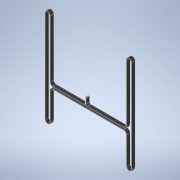
# Autodesk Inventor part: GT2 Belt
Saved by Autodesk Inventor 2022 (Build 260153000, 153)
## iProperties
Created: 2022-06-12
Part Number: GT2 Belt
Material: Generic
Document SubType Name: Modeling
Designer: Nick
Density: 1 g/cm^3
Appearance: Default
Author: Nick
Autodesk Inventor part; units mm, degrees
ref_plane "YZ Plane" through (0, 0, 0) normal (1, 0, 0) x (0, 1, 0)
ref_plane "Work Plane1" through (-134.6469, -237.4299, -822.9431) normal (0, 0, -1) x (0, -1, 0)
ref_plane "Work Plane3" through (-210.2684, -168.4601, -822.9431) normal (0, 1, 0) x (-1, 0, 0)
sketch "Sketch3" plane through (-210.2684, -168.4601, -822.9431) normal (0, 1, 0) x (-1, 0, 0)
  line L0 (0, 0) -> (1, 0)
  line L1 (1, 0) -> (1, -6)
  line L2 (1, -6) -> (0, -6)
  line L3 (0, -6) -> (0, 0)
  point P0 (-210.2684, 822.9431)
  dimension "d10" = 1
  dimension "d11" = 6
  constraints: 8 end point, 2 parallel, 1 horizontal, 1 perpendicular
  measures "d10" distance of L1.end L2.end
  measures "d11" distance of L0.end L1.end
sketch "Sketch1" plane through (-134.6469, -237.4299, -822.9431) normal (0, 0, -1) x (0, -1, 0)
  line L0 (0, 4.84) -> (-47.9698, 4.84)
  line L1 (-52.6298, 9.5) -> (-52.6298, 134.5)
  line L2 (-57.3098, 134.5) -> (-57.3098, 79.9614)
  line L3 (-57.3098, 73.4614) -> (-57.3098, 9.5)
  line L4 (-163, 4.84) -> (-61.9698, 4.84)
  line L5 (-163, -4.84) -> (0, -4.84)
  circle A0 centre (-61.9698, 9.5) radius 4.5 construction
  circle A1 centre (-47.9698, 9.5) radius 4.5 construction
  circle A2 centre (-61.9698, 134.5) radius 4.5
  circle A3 centre (-47.9698, 134.5) radius 4.5
  circle A4 centre (-163, 0) radius 4.5 construction
  circle A5 centre (-163, 144) radius 4.5
  arc A6 (1.9272, 148.2347) -> (2.8669, 147.6644) centre (2.3867, 147.9324) ccw construction
  arc A7 (3.1094, 147.709) -> (2.8669, 147.6644) centre (3.0067, 147.5864) ccw construction
  arc A8 (3.4244, 147.4203) -> (3.1094, 147.709) centre (0, 144) ccw construction
  arc A9 (3.4011, 147.1749) -> (3.4244, 147.4203) centre (3.3112, 147.3073) ccw construction
  arc A10 (3.4011, 147.1749) -> (4.051, 146.2883) centre (3.7099, 146.7197) ccw construction
  arc A11 (4.2921, 146.2368) -> (4.051, 146.2883) centre (4.1503, 146.1628) ccw construction
  arc A12 (4.4727, 145.8495) -> (4.2921, 146.2368) centre (0, 144) ccw construction
  arc A13 (4.3571, 145.6317) -> (4.4727, 145.8495) centre (4.3248, 145.7884) ccw construction
  arc A14 (4.3571, 145.6317) -> (4.6183, 144.5639) centre (4.4683, 145.093) ccw construction
  arc A15 (4.8214, 144.424) -> (4.6183, 144.5639) centre (4.662, 144.41) ccw construction
  arc A16 (4.84, 143.9971) -> (4.8214, 144.424) centre (0, 144) ccw construction
  arc A17 (4.6499, 143.8401) -> (4.84, 143.9971) centre (4.68, 143.9972) ccw construction
  arc A18 (4.6499, 143.8401) -> (4.4826, 142.7536) centre (4.5464, 143.2999) ccw construction
  arc A19 (4.6166, 142.5466) -> (4.4826, 142.7536) centre (4.464, 142.5947) ccw construction
  arc A20 (4.4705, 142.1451) -> (4.6166, 142.5466) centre (0, 144) ccw construction
  arc A21 (4.2347, 142.0728) -> (4.4705, 142.1451) centre (4.3227, 142.2065) ccw construction
  arc A22 (4.2347, 142.0728) -> (3.6644, 141.1331) centre (3.9324, 141.6133) ccw construction
  arc A23 (3.709, 140.8906) -> (3.6644, 141.1331) centre (3.5864, 140.9933) ccw construction
  arc A24 (3.4203, 140.5756) -> (3.709, 140.8906) centre (0, 144) ccw construction
  arc A25 (3.1749, 140.5989) -> (3.4203, 140.5756) centre (3.3073, 140.6888) ccw construction
  arc A26 (3.1749, 140.5989) -> (2.2883, 139.949) centre (2.7197, 140.2901) ccw construction
  arc A27 (2.2368, 139.7079) -> (2.2883, 139.949) centre (2.1628, 139.8497) ccw construction
  arc A28 (1.8495, 139.5273) -> (2.2368, 139.7079) centre (0, 144) ccw construction
  arc A29 (1.6317, 139.6429) -> (1.8495, 139.5273) centre (1.7884, 139.6752) ccw construction
  arc A30 (1.6317, 139.6429) -> (0.5639, 139.3817) centre (1.093, 139.5317) ccw construction
  arc A31 (0.424, 139.1786) -> (0.5639, 139.3817) centre (0.41, 139.338) ccw construction
  arc A32 (-0.0029, 139.16) -> (0.424, 139.1786) centre (0, 144) ccw construction
  arc A33 (-0.1599, 139.3501) -> (-0.0029, 139.16) centre (-0.0028, 139.32) ccw construction
  arc A34 (-0.1599, 139.3501) -> (-1.2464, 139.5174) centre (-0.7001, 139.4536) ccw construction
  arc A35 (-1.4534, 139.3834) -> (-1.2464, 139.5174) centre (-1.4053, 139.536) ccw construction
  arc A36 (-1.8549, 139.5295) -> (-1.4534, 139.3834) centre (0, 144) ccw construction
  arc A37 (-1.9272, 139.7653) -> (-1.8549, 139.5295) centre (-1.7935, 139.6773) ccw construction
  arc A38 (-1.9272, 139.7653) -> (-2.8669, 140.3356) centre (-2.3867, 140.0676) ccw construction
  arc A39 (-3.1094, 140.291) -> (-2.8669, 140.3356) centre (-3.0067, 140.4136) ccw construction
  arc A40 (-3.4244, 140.5797) -> (-3.1094, 140.291) centre (0, 144) ccw construction
  arc A41 (-3.4011, 140.8251) -> (-3.4244, 140.5797) centre (-3.3112, 140.6927) ccw construction
  arc A42 (-3.4011, 140.8251) -> (-4.051, 141.7117) centre (-3.7099, 141.2803) ccw construction
  arc A43 (-4.2921, 141.7632) -> (-4.051, 141.7117) centre (-4.1503, 141.8372) ccw construction
  arc A44 (-4.4727, 142.1505) -> (-4.2921, 141.7632) centre (0, 144) ccw construction
  arc A45 (-4.3571, 142.3683) -> (-4.4727, 142.1505) centre (-4.3248, 142.2116) ccw construction
  arc A46 (-4.3571, 142.3683) -> (-4.6183, 143.4361) centre (-4.4683, 142.907) ccw construction
  arc A47 (-4.8214, 143.576) -> (-4.6183, 143.4361) centre (-4.662, 143.59) ccw construction
  arc A48 (-4.84, 144.0029) -> (-4.8214, 143.576) centre (0, 144) ccw construction
  arc A49 (-4.6499, 144.1599) -> (-4.84, 144.0029) centre (-4.68, 144.0028) ccw construction
  arc A50 (-4.6499, 144.1599) -> (-4.4826, 145.2464) centre (-4.5464, 144.7001) ccw construction
  arc A51 (-4.6166, 145.4534) -> (-4.4826, 145.2464) centre (-4.464, 145.4053) ccw construction
  arc A52 (-4.4705, 145.8549) -> (-4.6166, 145.4534) centre (0, 144) ccw construction
  arc A53 (-4.2347, 145.9272) -> (-4.4705, 145.8549) centre (-4.3227, 145.7935) ccw construction
  arc A54 (-4.2347, 145.9272) -> (-3.6644, 146.8669) centre (-3.9324, 146.3867) ccw construction
  arc A55 (-3.709, 147.1094) -> (-3.6644, 146.8669) centre (-3.5864, 147.0067) ccw construction
  arc A56 (-3.4203, 147.4244) -> (-3.709, 147.1094) centre (0, 144) ccw construction
  arc A57 (-3.1749, 147.4011) -> (-3.4203, 147.4244) centre (-3.3073, 147.3112) ccw construction
  arc A58 (-3.1749, 147.4011) -> (-2.2883, 148.051) centre (-2.7197, 147.7099) ccw construction
  arc A59 (-2.2368, 148.2921) -> (-2.2883, 148.051) centre (-2.1628, 148.1503) ccw construction
  arc A60 (-1.8495, 148.4727) -> (-2.2368, 148.2921) centre (0, 144) ccw construction
  arc A61 (-1.6317, 148.3571) -> (-1.8495, 148.4727) centre (-1.7884, 148.3248) ccw construction
  arc A62 (-1.6317, 148.3571) -> (-0.5639, 148.6183) centre (-1.093, 148.4683) ccw construction
  arc A63 (-0.424, 148.8214) -> (-0.5639, 148.6183) centre (-0.41, 148.662) ccw construction
  arc A64 (0.0029, 148.84) -> (-0.424, 148.8214) centre (0, 144) ccw construction
  arc A65 (0.1599, 148.6499) -> (0.0029, 148.84) centre (0.0028, 148.68) ccw construction
  arc A66 (0.1599, 148.6499) -> (1.2464, 148.4826) centre (0.7001, 148.5464) ccw construction
  arc A67 (1.4534, 148.6166) -> (1.2464, 148.4826) centre (1.4053, 148.464) ccw construction
  arc A68 (1.8549, 148.4705) -> (1.4534, 148.6166) centre (0, 144) ccw construction
  arc A69 (1.9272, 148.2347) -> (1.8549, 148.4705) centre (1.7935, 148.3227) ccw construction
  arc A70 (3.6555, -2.8782) -> (2.8782, -3.6555) centre (3.2527, -3.2527) ccw construction
  arc A71 (2.864, -3.9017) -> (2.8782, -3.6555) centre (2.7693, -3.7727) ccw construction
  arc A72 (2.5087, -4.1391) -> (2.864, -3.9017) centre (0, 0) ccw construction
  arc A73 (2.2758, -4.058) -> (2.5087, -4.1391) centre (2.4258, -4.0023) ccw construction
  arc A74 (2.2758, -4.058) -> (1.2602, -4.4787) centre (1.7603, -4.2498) ccw construction
  arc A75 (1.1528, -4.7007) -> (1.2602, -4.4787) centre (1.1147, -4.5453) ccw construction
  arc A76 (0.7338, -4.7841) -> (1.1528, -4.7007) centre (0, 0) ccw construction
  arc A77 (0.5496, -4.6201) -> (0.7338, -4.7841) centre (0.7095, -4.6259) ccw construction
  arc A78 (0.5496, -4.6201) -> (-0.5496, -4.6201) centre (0, -4.6) ccw construction
  arc A79 (-0.7338, -4.7841) -> (-0.5496, -4.6201) centre (-0.7095, -4.6259) ccw construction
  arc A80 (-1.1528, -4.7007) -> (-0.7338, -4.7841) centre (0, 0) ccw construction
  arc A81 (-1.2602, -4.4787) -> (-1.1528, -4.7007) centre (-1.1147, -4.5453) ccw construction
  arc A82 (-1.2602, -4.4787) -> (-2.2758, -4.058) centre (-1.7603, -4.2498) ccw construction
  arc A83 (-2.5087, -4.1391) -> (-2.2758, -4.058) centre (-2.4258, -4.0023) ccw construction
  arc A84 (-2.864, -3.9017) -> (-2.5087, -4.1391) centre (0, 0) ccw construction
  arc A85 (-2.8782, -3.6555) -> (-2.864, -3.9017) centre (-2.7693, -3.7727) ccw construction
  arc A86 (-2.8782, -3.6555) -> (-3.6555, -2.8782) centre (-3.2527, -3.2527) ccw construction
  arc A87 (-3.9017, -2.864) -> (-3.6555, -2.8782) centre (-3.7727, -2.7693) ccw construction
  arc A88 (-4.1391, -2.5087) -> (-3.9017, -2.864) centre (0, 0) ccw construction
  arc A89 (-4.058, -2.2758) -> (-4.1391, -2.5087) centre (-4.0023, -2.4258) ccw construction
  arc A90 (-4.058, -2.2758) -> (-4.4787, -1.2602) centre (-4.2498, -1.7603) ccw construction
  arc A91 (-4.7007, -1.1528) -> (-4.4787, -1.2602) centre (-4.5453, -1.1147) ccw construction
  arc A92 (-4.7841, -0.7338) -> (-4.7007, -1.1528) centre (0, 0) ccw construction
  arc A93 (-4.6201, -0.5496) -> (-4.7841, -0.7338) centre (-4.6259, -0.7095) ccw construction
  arc A94 (-4.6201, -0.5496) -> (-4.6201, 0.5496) centre (-4.6, 0) ccw construction
  arc A95 (-4.7841, 0.7338) -> (-4.6201, 0.5496) centre (-4.6259, 0.7095) ccw construction
  arc A96 (-4.7007, 1.1528) -> (-4.7841, 0.7338) centre (0, 0) ccw construction
  arc A97 (-4.4787, 1.2602) -> (-4.7007, 1.1528) centre (-4.5453, 1.1147) ccw construction
  arc A98 (-4.4787, 1.2602) -> (-4.058, 2.2758) centre (-4.2498, 1.7603) ccw construction
  arc A99 (-4.1391, 2.5087) -> (-4.058, 2.2758) centre (-4.0023, 2.4258) ccw construction
  arc A100 (-3.9017, 2.864) -> (-4.1391, 2.5087) centre (0, 0) ccw construction
  arc A101 (-3.6555, 2.8782) -> (-3.9017, 2.864) centre (-3.7727, 2.7693) ccw construction
  arc A102 (-3.6555, 2.8782) -> (-2.8782, 3.6555) centre (-3.2527, 3.2527) ccw construction
  arc A103 (-2.864, 3.9017) -> (-2.8782, 3.6555) centre (-2.7693, 3.7727) ccw construction
  arc A104 (-2.5087, 4.1391) -> (-2.864, 3.9017) centre (0, 0) ccw construction
  arc A105 (-2.2758, 4.058) -> (-2.5087, 4.1391) centre (-2.4258, 4.0023) ccw construction
  arc A106 (-2.2758, 4.058) -> (-1.2602, 4.4787) centre (-1.7603, 4.2498) ccw construction
  arc A107 (-1.1528, 4.7007) -> (-1.2602, 4.4787) centre (-1.1147, 4.5453) ccw construction
  arc A108 (-0.7338, 4.7841) -> (-1.1528, 4.7007) centre (0, 0) ccw construction
  arc A109 (-0.5496, 4.6201) -> (-0.7338, 4.7841) centre (-0.7095, 4.6259) ccw construction
  arc A110 (-0.5496, 4.6201) -> (0.5496, 4.6201) centre (0, 4.6) ccw construction
  arc A111 (0.7338, 4.7841) -> (0.5496, 4.6201) centre (0.7095, 4.6259) ccw construction
  arc A112 (1.1528, 4.7007) -> (0.7338, 4.7841) centre (0, 0) ccw construction
  arc A113 (1.2602, 4.4787) -> (1.1528, 4.7007) centre (1.1147, 4.5453) ccw construction
  arc A114 (1.2602, 4.4787) -> (2.2758, 4.058) centre (1.7603, 4.2498) ccw construction
  arc A115 (2.5087, 4.1391) -> (2.2758, 4.058) centre (2.4258, 4.0023) ccw construction
  arc A116 (2.864, 3.9017) -> (2.5087, 4.1391) centre (0, 0) ccw construction
  arc A117 (2.8782, 3.6555) -> (2.864, 3.9017) centre (2.7693, 3.7727) ccw construction
  arc A118 (2.8782, 3.6555) -> (3.6555, 2.8782) centre (3.2527, 3.2527) ccw construction
  arc A119 (3.9017, 2.864) -> (3.6555, 2.8782) centre (3.7727, 2.7693) ccw construction
  arc A120 (4.1391, 2.5087) -> (3.9017, 2.864) centre (0, 0) ccw construction
  arc A121 (4.058, 2.2758) -> (4.1391, 2.5087) centre (4.0023, 2.4258) ccw construction
  arc A122 (4.058, 2.2758) -> (4.4787, 1.2602) centre (4.2498, 1.7603) ccw construction
  arc A123 (4.7007, 1.1528) -> (4.4787, 1.2602) centre (4.5453, 1.1147) ccw construction
  arc A124 (4.7841, 0.7338) -> (4.7007, 1.1528) centre (0, 0) ccw construction
  arc A125 (4.6201, 0.5496) -> (4.7841, 0.7338) centre (4.6259, 0.7095) ccw construction
  arc A126 (4.6201, 0.5496) -> (4.6201, -0.5496) centre (4.6, 0) ccw construction
  arc A127 (4.7841, -0.7338) -> (4.6201, -0.5496) centre (4.6259, -0.7095) ccw construction
  arc A128 (4.7007, -1.1528) -> (4.7841, -0.7338) centre (0, 0) ccw construction
  arc A129 (4.4787, -1.2602) -> (4.7007, -1.1528) centre (4.5453, -1.1147) ccw construction
  arc A130 (4.4787, -1.2602) -> (4.058, -2.2758) centre (4.2498, -1.7603) ccw construction
  arc A131 (4.1391, -2.5087) -> (4.058, -2.2758) centre (4.0023, -2.4258) ccw construction
  arc A132 (3.9017, -2.864) -> (4.1391, -2.5087) centre (0, 0) ccw construction
  arc A133 (3.6555, -2.8782) -> (3.9017, -2.864) centre (3.7727, -2.7693) ccw construction
  arc A134 (-47.9698, 139.16) -> (-52.6298, 134.5) centre (-47.9698, 134.5) ccw
  arc A135 (-57.3098, 134.5) -> (-61.9698, 139.16) centre (-61.9698, 134.5) ccw
  arc A136 (-163, 148.84) -> (-163, 139.16) centre (-163, 144) ccw
  line L6 (-163, 139.16) -> (-61.9698, 139.16)
  arc A137 (-52.6298, 9.5) -> (-47.9698, 4.84) centre (-47.9698, 9.5) ccw
  arc A138 (-61.9698, 4.84) -> (-57.3098, 9.5) centre (-61.9698, 9.5) ccw
  arc A139 (-163, 4.84) -> (-163, -4.84) centre (-163, 0) ccw
  line L7 (-57.4698, 82.7114) -> (-51.4698, 82.7114) construction
  line L8 (-57.4698, 79.9614) -> (-57.4698, 82.7114) construction
  arc A140 (-59.4698, 77.9614) -> (-57.4698, 79.9614) centre (-59.4698, 79.9614) ccw construction
  line L9 (-68.9698, 77.9614) -> (-59.4698, 77.9614) construction
  line L10 (-68.9698, 75.4614) -> (-68.9698, 77.9614) construction
  line L11 (-59.4698, 75.4614) -> (-68.9698, 75.4614) construction
  arc A141 (-57.4698, 73.4614) -> (-59.4698, 75.4614) centre (-59.4698, 73.4614) ccw construction
  line L12 (-57.4698, 70.7114) -> (-57.4698, 73.4614) construction
  line L13 (-51.4698, 70.7114) -> (-57.4698, 70.7114) construction
  line L14 (-51.4698, 82.7114) -> (-51.4698, 70.7114) construction
  arc A142 (-57.3098, 73.4614) -> (-59.4698, 75.6214) centre (-59.4698, 73.4614) ccw
  arc A143 (-59.4698, 77.8014) -> (-57.3098, 79.9614) centre (-59.4698, 79.9614) ccw
  line L15 (-59.4698, 75.6214) -> (-68.9698, 75.6214)
  line L16 (-59.4698, 77.8014) -> (-68.9698, 77.8014)
  line L17 (-47.9698, 139.16) -> (0, 139.16)
  line L18 (0, 148.84) -> (-163, 148.84)
  arc A144 (0, 139.16) -> (0, 148.84) centre (0, 144) ccw
  arc A145 (0, -4.84) -> (0, 4.84) centre (0, 0) ccw
  point P0 (-237.4299, -134.6469)
sweep "Sweep3" add profiles "Sketch3" path "Sketch1" path curves L15 A142 L3 A138 L4 A139 L5 A145 L0 A137 L1 A134 L17 A144 L18 A136 L6 A135 L2 A143 L16
body "Solid4"
